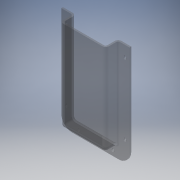
# Autodesk Inventor part: M178-4001-03
Saved by Autodesk Inventor 2018 (Build 220105000, 105)
## iProperties
Created: 2004-11-29
Part Number: M178-4001-03
Material: Plastic, Clear
Document SubType Name: Modeling
Designer: Autodesk, Inc.
Manufacturer: Standard
Standards Organization: Custom
Description: TOOL CADDY, PLASTIC, 2 x 4 x 0.625
Mass: 26.1813 g
Surface Area: 237.698 cm^2
Volume: 21.8178 cm^3
Density: 1.2 g/cm^3
Appearance: Plastic (Clear)
CAGE: 1LJX3
Dept. ID: Product Design
Description #2: ---
Finish #1: ---
Finish #2: ---
Material ID: ---
Project Number: ---
Author: Autodesk, Inc.
Autodesk Inventor part; units mm, degrees
ref_plane "YZ Plane" through (0, 0, 0) normal (1, 0, 0) x (0, 1, 0)
ref_plane "XZ Plane" through (0, 0, 0) normal (0, 1, 0) x (-1, 0, 0)
ref_plane "XY Plane" through (0, 0, 0) normal (0, 0, 1) x (1, 0, 0)
sketch "Sketch1" plane through (0, 0, 0) normal (0, 0, 1) x (1, 0, 0)
  line L0 (-25.4, 50.8) -> (25.4, 50.8)
  line L1 (25.4, 50.8) -> (25.4, -50.8)
  line L2 (25.4, -50.8) -> (-25.4, -50.8)
  line L3 (-25.4, -50.8) -> (-25.4, 50.8)
  point P0 (0, 0)
  point P1 (0, 50.8)
  point P2 (-25.4, 0)
  dimension "Width" = 50.8
  dimension "Height" = 101.6
  constraints: 8 end point, 2 midpoint, 2 parallel, 1 horizontal, 1 horizontal alignment, 1 perpendicular, 1 vertical alignment
  measures "Width" distance of L1.end L2.end
  measures "Height" distance of L2.end L0.start
extrude "Extrusion1" add sketch "Sketch1" along normal blind 15.875
shell "Shell1" thickness 1.905 removed faces 2 at (-8.4667, 50.8, 5.2917) at (-8.4667, 16.9333, 0)
sketch "Sketch2" plane through (0, 0, 0) normal (0, 0, -1) x (-1, 0, 0)
  line L0 (-25.4, 50.8) -> (-25.4, -50.8) projected
  line L1 (25.4, -50.8) -> (25.4, 50.8) projected
  line L2 (-25.4, -50.8) -> (25.4, -50.8) projected
  line L3 (25.4, 50.8) -> (38.1, 50.8)
  line L4 (38.1, 50.8) -> (38.1, -51.435)
  arc A0 (26.035, -63.5) -> (38.1, -51.435) centre (26.035, -51.435) ccw
  line L5 (26.035, -63.5) -> (-26.035, -63.5)
  arc A1 (-38.1, -51.435) -> (-26.035, -63.5) centre (-26.035, -51.435) ccw
  line L6 (-38.1, -51.435) -> (-38.1, 50.8)
  line L7 (-38.1, 50.8) -> (-25.4, 50.8)
  dimension "d5" = 12.7
  dimension "d6" = 12.7
  dimension "d7" = 12.065
  constraints: 10 end point, 4 point on circle, 4 tangent, 3 parallel, 2 centre point, 2 collinear, 1 equal radius, 1 perpendicular
  measures "d5" distance of L6.end L0.start
  measures "d6" distance between parallel lines of L2 L5
  measures "d7" radius of A1
extrude "Extrusion2" add sketch "Sketch2" against normal blind 1.905
fillet "Fillet1" radius 1.905 8 edges at (23.495, 0.9525, 13.97) (0, -48.895, 13.97) (23.495, -48.895, 6.985) (-23.495, -48.895, 6.985) (-23.495, 0.9525, 13.97) (-25.4, 0, 1.905) (0, -50.8, 1.905) (25.4, 0, 1.905)
fillet "Fillet1" radius 3.81 8 edges at (0, -50.8, 15.875) (25.4, 0, 15.875) (-25.4, 0, 15.875) (-25.4, -50.8, 8.89) (25.4, -50.8, 8.89) (-23.495, 0.9525, 0) (0, -48.895, 0) (23.495, 0.9525, 0)
sketch "Sketch3" plane through (0, 0, 0) normal (0, 0, -1) x (-1, 0, 0)
  line L0 (-27.305, 50.8) -> (-38.1, 50.8) projected
  arc A0 (-38.1, -51.435) -> (-26.035, -63.5) centre (-26.035, -51.435) ccw projected
  line L1 (-38.1, -51.435) -> (-38.1, 50.8) projected
  line L2 (26.035, -63.5) -> (-26.035, -63.5) projected
  line L3 (0, -63.5) -> (0, -52.705) construction
  line L4 (-21.59, -52.705) -> (21.59, -52.705) construction
  line L5 (0, -89.3585) -> (0, 74.1597) construction
  point P0 (-32.7025, 38.1)
  point P1 (-32.7025, -41.275)
  point P2 (-19.05, -58.1025)
  point P3 (-32.7025, 50.8)
  point P4 (-32.7025, 50.8)
  point P5 (0, -58.1025)
  point P6 (32.7025, 38.1)
  point P7 (32.7025, -41.275)
  point P8 (19.05, -58.1025)
  dimension "d13" = 19.05
  dimension "d14" = 22.225
  dimension "d15" = 12.7
  constraints: 5 midpoint, 3 symmetric about line, 2 end point, 2 vertical alignment, 1 horizontal alignment, 1 perpendicular
  measures "d13" distance from line of point (-19.05, -58.102) L1
  measures "d14" distance from line of point (-32.702, -41.275) L2
  measures "d15" distance from line of point (-32.702, 38.1) L0
hole "Hole1" at (32.7025, 38.1, 0) at (32.7025, -41.275, 0) at (19.05, -58.1025, 0) at (-32.7025, 38.1, 0) at (-32.7025, -41.275, 0) at (-19.05, -58.1025, 0) direction (0, 0, 1) diameter 3.175 end through all clearance for "Flat Head Machine Screw (82)" size "#4" standard "Ansi Unified Screw Threads"
body "Solid1"
